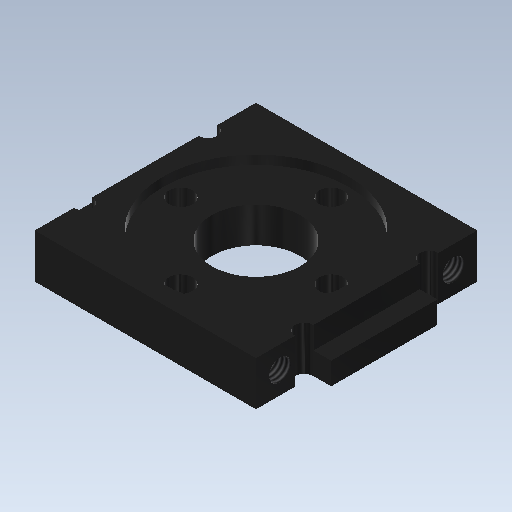
# Autodesk Inventor part: Head_horizontal_frame_01
Saved by Autodesk Inventor 2020.4 (Build 244396000, 396)
## iProperties
Created: 2016-05-04
Part Number: Head_horizontal_frame_01
Material: アセタール樹脂、黒
Document SubType Name: Modeling
Designer: hiroaki
Density: 1.425 g/cm^3
Appearance: 滑らか - 黒
Mass: 5.91414 g
Surface Area: 28.2108 cm^2
Volume: 4.15027 cm^3
Description: POM T5
Category: 頭
d0: 25.000 mm
d1: 1.050 mm
d3: 6.500 mm
d4: 3.100 mm
d6: 4.000 mm
d14: 5.000 mm
d15: 0.00 deg
d17: 5.000 mm
d18: 2.700 mm
d21: 6.000 mm
d25: 8.800 mm
d27: 2.000 ul
d28: 360.00 deg
Author: hiroaki
Autodesk Inventor part; units mm, degrees
ref_plane "YZ Plane" through (0, 0, 0) normal (1, 0, 0) x (0, 1, 0)
ref_plane "XZ Plane" through (0, 0, 0) normal (0, 1, 0) x (-1, 0, 0)
ref_plane "XY Plane" through (0, 0, 0) normal (0, 0, 1) x (1, 0, 0)
sketch "スケッチ1" plane through (0, 0, 0) normal (0, 0, 1) x (1, 0, 0)
  line L0 (12.5, -12.5) -> (12.5, 12.5) construction
  line L1 (-12.5, 12.5) -> (-12.5, -12.5) construction
  line L2 (-12.5, -12.5) -> (12.5, 12.5) construction
  line L3 (12.5, -12.5) -> (-12.5, 12.5) construction
  line L4 (-8.1, 12.5) -> (-12.5, 12.5)
  line L5 (-12.5, 12.5) -> (-12.5, 8.9019)
  line L6 (8.1, 12.5) -> (12.5, 12.5)
  line L7 (12.5, 12.5) -> (12.5, 8.1)
  line L8 (-12.5, -7.2981) -> (-12.5, -12.5)
  line L9 (-12.5, -12.5) -> (-8.1, -12.5)
  line L10 (8.1, -12.5) -> (12.5, -12.5)
  line L11 (12.5, -12.5) -> (12.5, -8.1)
  line L12 (-6, 12.5) -> (-6, 14.5)
  line L13 (-6, 14.5) -> (6, 14.5)
  line L14 (6, 14.5) -> (6, 12.5)
  arc A0 (-8.1, 12.5) -> (-6, 12.5) centre (-7.05, 12.5) ccw
  arc A1 (6, 12.5) -> (8.1, 12.5) centre (7.05, 12.5) ccw
  line L15 (0, 12.5) -> (0, 0) construction
  line L16 (0, 0) -> (12.5, 0) construction
  line L17 (-6, -12.5) -> (-6, -14.5)
  line L18 (-6, -14.5) -> (6, -14.5)
  line L19 (6, -14.5) -> (6, -12.5)
  arc A2 (-6, -12.5) -> (-8.1, -12.5) centre (-7.05, -12.5) ccw
  arc A3 (8.1, -12.5) -> (6, -12.5) centre (7.05, -12.5) ccw
  line L20 (-11.35, 12.5) -> (-8.25, 12.5) construction
  line L21 (-8.25, 12.5) -> (-8.25, 8.5) construction
  line L22 (-8.25, 8.5) -> (-11.35, 8.5) construction
  line L23 (-11.35, 8.5) -> (-11.35, 12.5) construction
  line L24 (-12.5, 6.7519) -> (-12.5, 9.8519) construction
  line L25 (-9.8, 12.5) -> (-9.8, 8.5) construction
  line L26 (-12.5, -12.5) -> (-12.5, 12.5)
  line L27 (12.5, -12.5) -> (12.5, 12.5)
  line L28 (0, -14.5) -> (0, 14.5) construction
  circle A4 centre (0, -8.5) radius 1.35
  circle A5 centre (8.5, 0) radius 1.35
  circle A6 centre (0, 8.5) radius 1.35
  circle A7 centre (-8.5, 0) radius 1.35
  circle A8 centre (0, 0) radius 5.01
  circle A9 centre (0, 0) radius 10.51
  line L29 (-6, 12.5) -> (6, 12.5)
  line L30 (-6, -12.5) -> (6, -12.5)
  dimension "d0" = 25
  dimension "d1" = 1.05
  dimension "d3" = 6.5
  dimension "d4" = 3.1
  dimension "d6" = 4
  dimension "d18" = 2.7
  dimension "d46" = 25
  dimension "d58" = 2.7
  dimension "d59" = 8.5
  dimension "d62" = 360
  dimension "d64" = 10.02
  dimension "d65" = 21.02
  dimension "d68" = 2
  constraints: 62 end point, 10 centre point, 9 perpendicular, 8 point on circle, 7 midpoint, 5 parallel, 4 collinear, 4 horizontal, 4 horizontal alignment, 4 symmetric about line, 4 tangent, 4 vertical, 2 coincident, 2 equal radius, 2 point on line, 13 other
  measures "d0" distance of L1.start L1.end
  measures "d1" radius of A0
  measures "d3" distance between parallel lines of L1 L12
  measures "d4" distance of L20.start L20.end
  measures "d6" distance between parallel lines of L4 L22
  measures "d18" distance between parallel lines of L5 L25
  measures "d46" distance of L0.end L1.start
  measures "d58" diameter of A4
  measures "d59" distance of L15.end A4.centre
  measures "d64" diameter of A8
  measures "d65" diameter of A9
  measures "d68" vertical distance of L1.start L12.end
extrude "押し出し1" add sketch "スケッチ1" along normal blind 5 contours A0 L29 A1 L6 L7 L27 L11 L10 A3 L30 A2 L9 L8 L26 L5 L4
sketch "スケッチ2" plane through (-12.5, -12.5, 5) normal (0, -1, 0) x (1, 0, 0)
  line L0 (12.5, 0) -> (12.5, -5.2657) construction
  line L1 (0, -2.5) -> (22.3, -2.5) construction
  line L2 (25, -5) -> (25, 0) projected
  line L3 (0, -5) -> (0, 0) projected
  line L4 (0, 0) -> (4.4, 0) projected
  point P0 (12.5, -5)
  point P1 (2.7, -2.5)
  dimension "d56" = 2.7
  dimension "d57" = 2.7
  dimension "d69" = 2.5
  constraints: 4 end point, 1 horizontal, 1 horizontal alignment, 1 midpoint, 1 symmetric about line, 1 vertical
  measures "d56" horizontal distance of L3.end point (2.7, -2.5)
  measures "d57" distance from line of L1.end L2
  measures "d69" distance from line of L1.start L4
hole "穴1" at (-9.8, -12.5, 2.5) at (9.8, -12.5, 2.5) direction (0, 1, 0) diameter 2.459 depth 8.8 thread size "M3x0.5" class "6H" standard "ISO Metric profile"
pattern_circular "円形状パターン1" count 2 over 360 about axis through (0, 0, -10) along (0, 0, 1) of "穴1"
extrude "押し出し2" add sketch "スケッチ1" along normal blind 4 contours A9
extrude "押し出し3" add sketch "スケッチ1" along normal blind 2.5 contours L12 L13 L14 L29 | L30 L19 L18 L17
equation "\"d57\" = d56"
